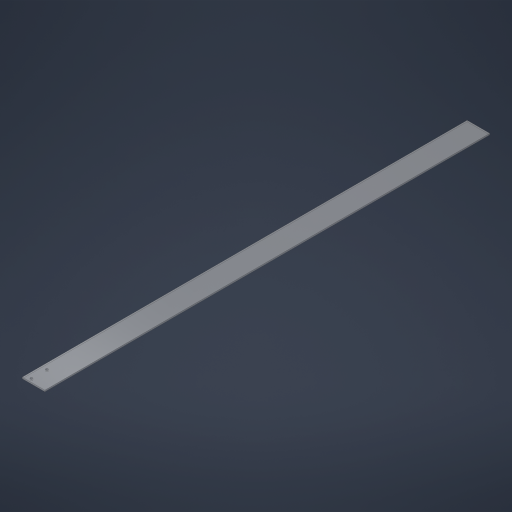
# Autodesk Inventor part: EL2-023
Saved by Autodesk Inventor 2023.4 (Build 274418000, 418)
## iProperties
Created: 2025-02-10
Part Number: EL2-023
Material: Polycarbonate, Clear
Document SubType Name: Sheet Metal
Designer: brand
Density: 1.2 g/cm^3
Sheet Metal Rule: Default
Appearance: Polycarbonate - Clear
Author: brand
Autodesk Inventor part; units mm, degrees
ref_plane "YZ Plane" through (0, 0, 0) normal (1, 0, 0) x (0, 1, 0)
ref_plane "XZ Plane" through (0, 0, 0) normal (0, 1, 0) x (-1, 0, 0)
ref_plane "XY Plane" through (0, 0, 0) normal (0, 0, 1) x (1, 0, 0)
sketch "Sketch1" plane through (0, 0, 0) normal (0, 1, 0) x (-1, 0, 0)
  line L0 (25.4, 500.0625) -> (-25.4, 500.0625)
  line L1 (-25.4, 500.0625) -> (-25.4, -500.0625)
  line L2 (-25.4, -500.0625) -> (25.4, -500.0625)
  line L3 (25.4, -500.0625) -> (25.4, 500.0625)
  line L4 (25.4, 500.0625) -> (-25.4, -500.0625) construction
  line L5 (-25.4, 500.0625) -> (25.4, -500.0625) construction
  point P0 (0, 0)
  dimension "d0" = 50.8
  dimension "d1" = 1000.125
  measures "d0" distance of L2.end L1.end
  measures "d1" distance of L1.end L0.end
extrude "Plate1" add sketch "Sketch1" along normal mid plane 3.175
sketch "Sketch2" plane through (0, 1.5875, 0) normal (0, 1, 0) x (1, 0, 0)
  line L0 (-25.4, -500.0625) -> (-25.4, 500.0625) construction
  line L1 (-25.4, 500.0625) -> (25.4, 500.0625) construction
  line L2 (25.4, 500.0625) -> (25.4, -500.0625) construction
  line L3 (25.4, -500.0625) -> (-25.4, -500.0625) construction
  point P0 (0, 0)
  point P1 (-12.7, -492.125)
  point P2 (-12.7, -457.2)
  dimension "d3" = 7.9375
  dimension "d4" = 34.925
  dimension "d5" = 12.7
  constraints: 1 vertical alignment
  measures "d3" distance from line of L3 point (-12.7, -492.125)
  measures "d4" distance of point (-12.7, -492.125) point (-12.7, -457.2)
  measures "d5" distance from line of point (-12.7, -492.125) L0
hole "Hole1" at (-12.7, 1.5875, 492.125) at (-12.7, 1.5875, 457.2) direction (0, -1, 0) diameter 5.1054 end through all clearance for "Flat Head Machine Screw (82)" size "#10" standard "Ansi Unified Screw Threads"
equation "\"d11\" = Thickness"
equation "\"d2\" = Thickness"
equation "\"BendRadius\" = Thickness"
equation "\"BendReliefWidth\" = Thickness"
equation "\"BendReliefDepth\" = 0.5 * Thickness"
equation "\"CornerReliefSize\" = 4 * Thickness"
equation "\"MinimumRemnant\" = 2 * Thickness"
equation "\"TransitionRadius\" = BendRadius"
equation "\"JacobiRadiusSize\" = BendRadius"
equation "\"GapSize\" = Thickness"
equation "\"Thickness\" = 3.175"
body "Solid1"
